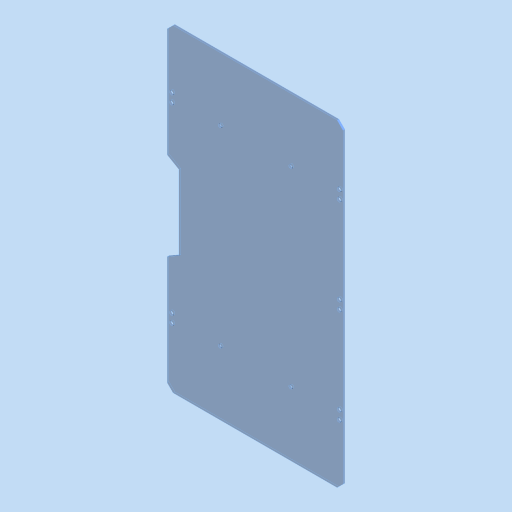
# Autodesk Inventor part: enc-BackPanel Unten HF-Durchlass
Saved by Autodesk Inventor 2023.2 (Build 272271000, 271)
## iProperties
Created: 2023-12-04
Part Number: enc-BackPanel Unten HF-Durchlass
Material: Generisch
Document SubType Name: Modeling
Designer: Nils Bade
Density: 1 g/cm^3
Appearance: PVC Verglasung
Description: Fertigung
Auf Bestellliste: True
Author: Nils Bade
Autodesk Inventor part; units mm, degrees
ref_plane "YZ Plane" through (0, 0, 0) normal (1, 0, 0) x (0, 1, 0)
ref_plane "XZ Plane" through (0, 0, 0) normal (0, 1, 0) x (-1, 0, 0)
ref_plane "XY Plane" through (0, 0, 0) normal (0, 0, 1) x (1, 0, 0)
sketch "Skizze1" plane through (0, 0, 0) normal (0, 0, 1) x (1, 0, 0)
  line L0 (-149.5, 270.5) -> (149.5, 270.5)
  line L1 (149.5, 270.5) -> (149.5, -270.5)
  line L2 (149.5, -270.5) -> (-149.5, -270.5)
  line L3 (-149.5, -270.5) -> (-149.5, 270.5)
  line L4 (-149.5, 270.5) -> (149.5, -270.5) construction
  line L5 (149.5, 270.5) -> (-149.5, -270.5) construction
  line L6 (-74.75, 270.5) -> (-74.75, -270.5) construction
  line L7 (0, 396.7) -> (0, -381.7) construction
  line L8 (-142.5, 270.5) -> (-142.5, -270.5) construction
  line L9 (-149.5, -162.3) -> (149.5, -162.3) construction
  circle A0 centre (-142.5, -154.8) radius 3.25
  circle A1 centre (-142.5, -169.8) radius 3.25
  line L10 (-222.3, 0) -> (287.3, 0) construction
  circle A2 centre (-142.5, 7.5) radius 3.25
  circle A3 centre (-142.5, -7.5) radius 3.25
  circle A4 centre (-142.5, 154.8) radius 3.25
  circle A5 centre (-142.5, 169.8) radius 3.25
  circle A6 centre (142.5, -154.8) radius 3.25
  circle A7 centre (142.5, -169.8) radius 3.25
  circle A8 centre (142.5, 7.5) radius 3.25
  circle A9 centre (142.5, -7.5) radius 3.25
  circle A10 centre (142.5, 169.8) radius 3.25
  circle A11 centre (142.5, 154.8) radius 3.25
  circle A12 centre (-60, -162.3) radius 2.75
  circle A13 centre (60, -162.3) radius 2.75
  circle A14 centre (-60, 162.3) radius 2.75
  circle A15 centre (60, 162.3) radius 2.75
  line L11 (214.5, 285.5) -> (84.5, 285.5) construction
  line L12 (84.5, 285.5) -> (84.5, 255.5)
  line L13 (84.5, 255.5) -> (214.5, 255.5)
  line L14 (214.5, 255.5) -> (214.5, 285.5) construction
  line L15 (214.5, 285.5) -> (84.5, 255.5) construction
  line L16 (84.5, 285.5) -> (214.5, 255.5) construction
  point P0 (0, 0)
  dimension "d0" = 541
  dimension "d1" = 299
  dimension "d2" = 74.75
  dimension "d3" = 7
  dimension "d4" = 108.2
  dimension "d5" = 6.5
  dimension "d6" = 7.5
  dimension "d7" = 6.5
  dimension "d8" = 7.5
  dimension "d9" = 7.5
  dimension "d10" = 6.5
  dimension "d11" = 5.5
  dimension "d12" = 60
  dimension "d15" = 130
  dimension "d16" = 15
  constraints: 30 end point, 16 centre point, 12 symmetric about line, 8 point on line, 4 midpoint, 4 parallel, 4 perpendicular, 2 horizontal, 1 vertical, 12 other
  measures "d0" distance of L0.end L1.end
  measures "d1" distance of L1.end L2.end
  measures "d2" distance between parallel lines of L3 L6
  measures "d3" distance between parallel lines of L3 L8
  measures "d4" distance between parallel lines of L2 L9
  measures "d5" diameter of A0
  measures "d6" distance from line of L9 A0.centre
  measures "d7" diameter of A2
  measures "d8" distance from line of L10 A2.centre
  measures "d9" distance from line of L10 A3.centre
  measures "d10" diameter of A3
  measures "d11" diameter of A12
  measures "d12" distance from line of L7 A12.centre
  measures "d15" distance of L11.start L11.end
  measures "d16" distance between parallel lines of L0 L13
extrude "Extrusion1" add sketch "Skizze1" along normal blind 3
chamfer "Fase1" distance 10 angle 45 4 edges at (149.5, 270.5, 1.5) (149.5, -270.5, 1.5) (-149.5, -270.5, 1.5) (-149.5, 270.5, 1.5)
ref_plane "HF-Kabel-DurchlassPunkt" through (-139.5, -56.5, 0) normal (0, -1, 0) x (1, 0, 0)
sketch "S-AussparungHFKabel" plane through (0, 0, 3) normal (0, 0, 1) x (1, 0, 0)
  line L0 (209.3, -56.5) -> (-209.3, -56.5) construction
  line L1 (-149.5, 260.5) -> (-149.5, -260.5) projected
  line L2 (-149.5, -75) -> (-129.5, -63.453)
  line L3 (-129.5, -63.453) -> (-129.5, 63.453)
  line L4 (-129.5, 63.453) -> (-149.5, 75)
  line L5 (-129.5, 0) -> (-149.5, 0) construction
  line L6 (-215.9, 0) -> (210.4, 0) construction
  point P0 (0, 0)
  dimension "d21" = 60
  dimension "d22" = 20
  dimension "d23" = 150
  constraints: 8 end point, 2 midpoint, 2 point on line, 1 collinear, 1 perpendicular, 1 vertical, 1 other
  measures "d21" angle of L1 L4
  measures "d22" distance between parallel lines of L1 L3
  measures "d23" distance of L2.start L4.end
extrude "Ex-Kabelaussparung" cut sketch "S-AussparungHFKabel" against normal blind 10
equation "\"d2\" = 0.25 * d1"
equation "\"d4\" = 0.2 * d0"
equation "\"d7\" = d5"
equation "\"d8\" = d6"
equation "\"d9\" = d6"
equation "\"d10\" = d5"
